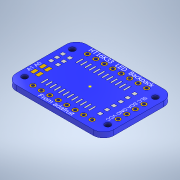
# Autodesk Inventor part: Part1
Saved by Autodesk Inventor 2021 (Build 250183000, 183)
## iProperties
Created: 2023-04-01
Part Number: Part1
Material: Generic
Document SubType Name: Modeling
Designer: stepa
Density: 1 g/cm^3
Appearance: Blue - Wall Paint - Glossy
Author: stepa
Autodesk Inventor part; units mm, degrees
ref_plane "YZ Plane" through (0, 0, 0) normal (1, 0, 0) x (0, 1, 0)
ref_plane "XZ Plane" through (0, 0, 0) normal (0, 1, 0) x (-1, 0, 0)
ref_plane "XY Plane" through (0, 0, 0) normal (0, 0, 1) x (1, 0, 0)
sketch "Sketch1" plane through (0, 0, 0) normal (0, 1, 0) x (-1, 0, 0)
  line L0 (11.15, -10.2) -> (-11.15, -10.2)
  line L1 (-14.15, -7.2) -> (-14.15, 7.2)
  line L2 (-11.15, 10.2) -> (11.15, 10.2)
  line L3 (14.15, 7.2) -> (14.15, -7.2)
  line L4 (14.15, -10.2) -> (-14.15, 10.2) construction
  line L5 (-14.15, -10.2) -> (14.15, 10.2) construction
  arc A0 (14.15, 7.2) -> (11.15, 10.2) centre (11.15, 7.2) ccw
  arc A1 (11.15, -10.2) -> (14.15, -7.2) centre (11.15, -7.2) ccw
  arc A2 (-14.15, -7.2) -> (-11.15, -10.2) centre (-11.15, -7.2) ccw
  arc A3 (-11.15, 10.2) -> (-14.15, 7.2) centre (-11.15, 7.2) ccw
  circle A4 centre (12.05, 6.9) radius 0.85
  circle A5 centre (12.05, -6.9) radius 0.85
  line L6 (0, 0) -> (0, 6.05)
  circle A6 centre (-12.05, 6.9) radius 0.85
  circle A7 centre (-12.05, -6.9) radius 0.85
  circle A8 centre (8.65, 7.9) radius 0.4
  circle A9 centre (6.2, 7.9) radius 0.4
  circle A10 centre (3.75, 7.9) radius 0.4
  circle A11 centre (1.3, 7.9) radius 0.4
  circle A12 centre (-1.15, 7.9) radius 0.4
  circle A13 centre (-3.6, 7.9) radius 0.4
  circle A14 centre (-6.05, 7.9) radius 0.4
  circle A15 centre (-8.5, 7.9) radius 0.4
  line L7 (0, 0) -> (3.75, 0)
  circle A16 centre (8.65, -7.9) radius 0.4
  circle A17 centre (6.2, -7.9) radius 0.4
  circle A18 centre (3.75, -7.9) radius 0.4
  circle A19 centre (1.3, -7.9) radius 0.4
  circle A20 centre (-1.15, -7.9) radius 0.4
  circle A21 centre (-3.6, -7.9) radius 0.4
  circle A22 centre (-6.05, -7.9) radius 0.4
  circle A23 centre (-8.5, -7.9) radius 0.4
  circle A24 centre (-12.15, 4) radius 0.4
  circle A25 centre (-12.15, 1.5) radius 0.4
  circle A26 centre (-12.15, -1) radius 0.4
  circle A27 centre (-12.15, -3.5) radius 0.4
  point P0 (0, -6.05)
  dimension "d0" = 20.4
  dimension "d1" = 28.3
  dimension "d2" = 3
  dimension "d3" = 1.7
  dimension "d4" = 1.7
  dimension "d5" = 3.3
  dimension "d6" = 3.3
  dimension "d7" = 2.1
  dimension "d8" = 2.1
  dimension "d9" = 0.8
  dimension "d10" = 5.5
  dimension "d11" = 2.3
  dimension "d14" = 2.45
  dimension "d19" = 0.8
  dimension "d20" = 2
  dimension "d21" = 2.5
  dimension "d22" = 6.2
  dimension "d23" = 0.8
  dimension "d24" = 2.5
  dimension "d25" = 0.8
  dimension "d26" = 0.8
  dimension "d27" = 2.5
  constraints: 28 centre point, 16 end point, 11 symmetric about line, 8 point on circle, 8 point on line, 8 tangent, 3 equal radius, 3 horizontal, 2 midpoint, 2 parallel, 1 perpendicular, 1 vertical, 24 other
  measures "d0" distance between parallel lines of L0 L2
  measures "d1" distance between parallel lines of L1 L3
  measures "d2" radius of A0
  measures "d3" diameter of A4
  measures "d4" diameter of A5
  measures "d5" distance from line of L0 A5.centre
  measures "d6" distance from line of L2 A4.centre
  measures "d7" distance from line of L3 A4.centre
  measures "d8" horizontal distance of L3.end A5.centre
  measures "d9" diameter of A8
  measures "d10" distance from line of L3 A8.centre
  measures "d11" distance from line of A8.centre L2
  measures "d14" distance of A8.centre A9.centre
  measures "d19" diameter of A24
  measures "d20" distance from line of L1 A24.centre
  measures "d21" distance of A24.centre A25.centre
  measures "d22" vertical distance of L2.start A24.centre
  measures "d23" diameter of A26
  measures "d24" distance of A25.centre A26.centre
  measures "d25" diameter of A27
  measures "d26" diameter of A25
  measures "d27" distance of A26.centre A27.centre
extrude "Extrusion1" add sketch "Sketch1" along normal mid plane 1.5
sketch "Sketch2" plane through (0, 0.75, 0) normal (0, 1, 0) x (1, 0, 0)
  line L0 (-11.15, -10.2) -> (11.15, -10.2) projected
  arc A0 (11.15, -10.2) -> (14.15, -7.2) centre (11.15, -7.2) ccw projected
  line L1 (14.15, -7.2) -> (14.15, 7.2) projected
  arc A1 (14.15, 7.2) -> (11.15, 10.2) centre (11.15, 7.2) ccw projected
  line L2 (11.15, 10.2) -> (-11.15, 10.2) projected
  arc A2 (-11.15, 10.2) -> (-14.15, 7.2) centre (-11.15, 7.2) ccw projected
  line L3 (-14.15, 7.2) -> (-14.15, -7.2) projected
  arc A3 (-14.15, -7.2) -> (-11.15, -10.2) centre (-11.15, -7.2) ccw projected
  circle A4 centre (12.15, 3.5) radius 0.4 projected
  circle A5 centre (12.15, -1.5) radius 0.4 projected
  circle A6 centre (3.6, 7.9) radius 0.4 projected
  circle A7 centre (6.05, 7.9) radius 0.4 projected
  circle A8 centre (-1.3, 7.9) radius 0.4 projected
  circle A9 centre (-6.2, 7.9) radius 0.4 projected
  circle A10 centre (8.5, -7.9) radius 0.4 projected
  circle A11 centre (6.05, -7.9) radius 0.4 projected
  circle A12 centre (3.6, -7.9) radius 0.4 projected
  circle A13 centre (1.15, -7.9) radius 0.4 projected
  circle A14 centre (-1.3, -7.9) radius 0.4 projected
  circle A15 centre (-3.75, -7.9) radius 0.4 projected
  circle A16 centre (-6.2, -7.9) radius 0.4 projected
  circle A17 centre (-8.65, -7.9) radius 0.4 projected
  circle A18 centre (-8.65, 7.9) radius 0.4 projected
  circle A19 centre (-3.75, 7.9) radius 0.4 projected
  circle A20 centre (1.15, 7.9) radius 0.4 projected
  circle A21 centre (8.5, 7.9) radius 0.4 projected
  circle A22 centre (12.15, -4) radius 0.4 projected
  circle A23 centre (12.15, 1) radius 0.4 projected
  circle A24 centre (12.05, 6.9) radius 0.85 projected
  circle A25 centre (12.05, -6.9) radius 0.85 projected
  circle A26 centre (-12.05, 6.9) radius 0.85 projected
  circle A27 centre (-12.05, -6.9) radius 0.85 projected
  circle A28 centre (-8.65, -7.9) radius 0.4 projected
  circle A29 centre (-8.65, -7.9) radius 0.75
  circle A30 centre (-6.2, -7.9) radius 0.4 projected
  circle A31 centre (-6.2, -7.9) radius 0.75
  circle A32 centre (-3.75, -7.9) radius 0.4 projected
  circle A33 centre (-3.75, -7.9) radius 0.75
  circle A34 centre (-1.3, -7.9) radius 0.4 projected
  circle A35 centre (-1.3, -7.9) radius 0.75
  circle A36 centre (1.15, -7.9) radius 0.4 projected
  circle A37 centre (1.15, -7.9) radius 0.75
  circle A38 centre (3.6, -7.9) radius 0.4 projected
  circle A39 centre (3.6, -7.9) radius 0.75
  circle A40 centre (6.05, -7.9) radius 0.4 projected
  circle A41 centre (6.05, -7.9) radius 0.75
  circle A42 centre (8.5, -7.9) radius 0.4 projected
  circle A43 centre (8.5, -7.9) radius 0.75
  circle A44 centre (12.15, -4) radius 0.4 projected
  circle A45 centre (12.15, -4) radius 0.75
  circle A46 centre (12.15, -1.5) radius 0.4 projected
  circle A47 centre (12.15, -1.5) radius 0.75
  circle A48 centre (12.15, 1) radius 0.4 projected
  circle A49 centre (12.15, 1) radius 0.75
  circle A50 centre (12.15, 3.5) radius 0.4 projected
  circle A51 centre (12.15, 3.5) radius 0.75
  circle A52 centre (8.5, 7.9) radius 0.4 projected
  circle A53 centre (8.5, 7.9) radius 0.75
  circle A54 centre (6.05, 7.9) radius 0.4 projected
  circle A55 centre (6.05, 7.9) radius 0.75
  circle A56 centre (3.6, 7.9) radius 0.4 projected
  circle A57 centre (3.6, 7.9) radius 0.75
  circle A58 centre (1.15, 7.9) radius 0.4 projected
  circle A59 centre (1.15, 7.9) radius 0.75
  circle A60 centre (-1.3, 7.9) radius 0.4 projected
  circle A61 centre (-1.3, 7.9) radius 0.75
  circle A62 centre (-3.75, 7.9) radius 0.4 projected
  circle A63 centre (-3.75, 7.9) radius 0.75
  circle A64 centre (-6.2, 7.9) radius 0.4 projected
  circle A65 centre (-6.2, 7.9) radius 0.75
  circle A66 centre (-8.65, 7.9) radius 0.75
  point P0 (0, 0)
  dimension "d30" = 1.5
  dimension "d31" = 1.5
  dimension "d32" = 1.5
  constraints: 20 centre point, 20 coincident
  measures "d30" diameter of A29
  measures "d31" diameter of A31
  measures "d32" diameter of A33
extrude "Extrusion2" cut sketch "Sketch2" against normal blind 0.001 contours A4 | A5 | A6 | A7 | A8 | A9 | A10 | A11 | A12 | A13 | A14 | A15 | A16 | A17 | A18 | A19 | A20 | A21 | A22 | A23 | A29 | A31 | A33 | A35 | A37 | A39 | A41 | A43 | A45 | A47 | A49 | A51 | A53 | A55 | A57 | A59 | A61 | A63 | A65 | A66
sketch "Sketch3" plane through (0, 0.75, 0) normal (0, 1, 0) x (1, 0, 0)
  line L0 (-12.55, -4.9) -> (-11.55, -4.9)
  line L1 (-11.55, -4.9) -> (-11.55, -3.3)
  line L2 (-11.55, -3.3) -> (-12.55, -3.3)
  line L3 (-12.55, -3.3) -> (-12.55, -4.9)
  line L4 (-12.55, -4.9) -> (-11.55, -3.3) construction
  line L5 (-11.55, -4.9) -> (-12.55, -3.3) construction
  line L6 (-14.15, 7.2) -> (-14.15, -7.2) projected
  line L7 (-11.15, -10.2) -> (11.15, -10.2) projected
  line L8 (-11.05, -4.9) -> (-10.05, -4.9)
  line L9 (-10.05, -4.9) -> (-10.05, -3.3)
  line L10 (-10.05, -3.3) -> (-11.05, -3.3)
  line L11 (-11.05, -3.3) -> (-11.05, -4.9)
  line L12 (-11.05, -4.9) -> (-10.05, -3.3) construction
  line L13 (-10.05, -4.9) -> (-11.05, -3.3) construction
  line L14 (-12.55, -2.4) -> (-11.55, -2.4)
  line L15 (-11.55, -2.4) -> (-11.55, -0.8)
  line L16 (-11.55, -0.8) -> (-12.55, -0.8)
  line L17 (-12.55, -0.8) -> (-12.55, -2.4)
  line L18 (-12.55, -2.4) -> (-11.55, -0.8) construction
  line L19 (-11.55, -2.4) -> (-12.55, -0.8) construction
  line L20 (-11.05, -2.4) -> (-10.05, -2.4)
  line L21 (-10.05, -2.4) -> (-10.05, -0.8)
  line L22 (-10.05, -0.8) -> (-11.05, -0.8)
  line L23 (-11.05, -0.8) -> (-11.05, -2.4)
  line L24 (-11.05, -2.4) -> (-10.05, -0.8) construction
  line L25 (-10.05, -2.4) -> (-11.05, -0.8) construction
  point P0 (0, 0)
  point P1 (-12.05, -4.1)
  point P2 (-10.55, -4.1)
  point P3 (-12.05, -1.6)
  point P4 (-10.55, -1.6)
  dimension "d35" = 1.6
  dimension "d36" = 1.6
  dimension "d37" = 1
  dimension "d38" = 5.3
  dimension "d41" = 1.5
  dimension "d44" = 2.5
  constraints: 48 end point, 8 midpoint, 2 collinear, 2 horizontal, 2 parallel, 1 perpendicular, 1 vertical, 31 other
  measures "d35" distance of L2.end L0.start
  measures "d36" distance between parallel lines of L6 L3
  measures "d37" distance of L1.end L2.end
  measures "d38" distance between parallel lines of L7 L0
  measures "d41" distance of L0.start L8.start
  measures "d44" distance of L0.start L14.start
extrude "Extrusion3" cut sketch "Sketch3" against normal blind 0.001
sketch "Sketch4" plane through (0, 0.75, 0) normal (0, 1, 0) x (1, 0, 0)
  line L0 (-5.456, -8.6683) -> (16.4652, -8.6683) construction
  line L1 (16.4652, -8.6683) -> (16.4652, 6.2441) construction
  line L2 (16.4652, 6.2441) -> (-5.456, 6.2441) construction
  line L3 (-5.456, 6.2441) -> (-5.456, -8.6683) construction
  line L4 (-13.845, -4.8059) -> (-13.845, 1.6171) construction
  line L5 (-13.845, 1.6171) -> (-10.9674, 1.6171) construction
  line L6 (-10.9674, 1.6171) -> (-10.9674, -4.8059) construction
  line L7 (-10.9674, -4.8059) -> (-13.845, -4.8059) construction
  line L8 (11.2525, 5.5942) -> (11.2525, -7.2168) construction
  line L9 (11.2525, -7.2168) -> (7.828, -7.2168) construction
  line L10 (7.828, -7.2168) -> (7.828, 5.5942) construction
  line L11 (7.828, 5.5942) -> (11.2525, 5.5942) construction
  line L12 (-9.4713, 10.0949) -> (13.4648, 10.0949) construction
  line L13 (13.4648, 10.0949) -> (13.4648, -4.2973) construction
  line L14 (13.4648, -4.2973) -> (-9.4713, -4.2973) construction
  line L15 (-9.4713, -4.2973) -> (-9.4713, 10.0949) construction
  point P0 (0, 0)
  dimension "d0" = 20.4
  dimension "d1" = 28.3
  dimension "d2" = 3
  dimension "d3" = 1.7
  dimension "d4" = 1.7
  dimension "d5" = 3.3
  dimension "d6" = 3.3
  dimension "d7" = 2.1
  dimension "d8" = 2.1
  dimension "d9" = 0.8
  dimension "d10" = 5.5
  dimension "d11" = 2.3
  dimension "d14" = 2.45
  dimension "d19" = 0.8
  dimension "d20" = 2
  dimension "d21" = 2.5
  dimension "d22" = 6.2
  dimension "d23" = 0.8
  dimension "d24" = 2.5
  dimension "d25" = 0.8
  dimension "d26" = 0.8
  dimension "d27" = 2.5
  constraints: 8 other
sketch "Sketch5" plane through (0, 0.75, 0) normal (0, 1, 0) x (1, 0, 0)
  line L0 (7.65, -5.7) -> (8.65, -5.7)
  line L1 (8.65, -5.7) -> (8.65, -4.7)
  line L2 (8.65, -4.7) -> (7.65, -4.7)
  line L3 (7.65, -4.7) -> (7.65, -5.7)
  line L4 (-11.15, -10.2) -> (11.15, -10.2) projected
  line L5 (14.15, -7.2) -> (14.15, 7.2) projected
  line L6 (7.65, -2.7) -> (7.65, -3.7)
  line L7 (7.65, -3.7) -> (8.65, -3.7)
  line L8 (8.65, -3.7) -> (8.65, -2.7)
  line L9 (8.65, -2.7) -> (7.65, -2.7)
  line L10 (7.65, 1.3) -> (7.65, 0.3)
  line L11 (7.65, -0.7) -> (7.65, -1.7)
  line L12 (7.65, 0.3) -> (8.65, 0.3)
  line L13 (7.65, -1.7) -> (8.65, -1.7)
  line L14 (8.65, 1.3) -> (7.65, 1.3)
  line L15 (8.65, -0.7) -> (7.65, -0.7)
  line L16 (8.65, -1.7) -> (8.65, -0.7)
  line L17 (8.65, 0.3) -> (8.65, 1.3)
  line L18 (7.65, 5.3) -> (7.65, 4.3)
  line L19 (7.65, 3.3) -> (7.65, 2.3)
  line L20 (7.65, 4.3) -> (8.65, 4.3)
  line L21 (7.65, 2.3) -> (8.65, 2.3)
  line L22 (8.65, 5.3) -> (7.65, 5.3)
  line L23 (8.65, 3.3) -> (7.65, 3.3)
  line L24 (8.65, 2.3) -> (8.65, 3.3)
  line L25 (8.65, 4.3) -> (8.65, 5.3)
  line L26 (-12.75, 0.4818) -> (-11.75, 0.4818)
  line L27 (-11.75, 0.4818) -> (-11.75, 1.4818)
  line L28 (-11.75, 1.4818) -> (-12.75, 1.4818)
  line L29 (-12.75, 1.4818) -> (-12.75, 0.4818)
  line L30 (-10.75, 0.4818) -> (-9.75, 0.4818)
  line L31 (-9.75, 0.4818) -> (-9.75, 1.4818)
  line L32 (-9.75, 1.4818) -> (-10.75, 1.4818)
  line L33 (-10.75, 1.4818) -> (-10.75, 0.4818)
  line L34 (-14.15, 7.2) -> (-14.15, -7.2) projected
  line L35 (-9.75, 2.1818) -> (-9.75, 3.1818)
  line L36 (-9.75, 3.1818) -> (-10.75, 3.1818)
  line L37 (-10.75, 2.1818) -> (-9.75, 2.1818)
  line L38 (-10.75, 3.1818) -> (-10.75, 2.1818)
  line L39 (-11.75, 2.1818) -> (-11.75, 3.1818)
  line L40 (-11.75, 3.1818) -> (-12.75, 3.1818)
  line L41 (-12.75, 2.1818) -> (-11.75, 2.1818)
  line L42 (-12.75, 3.1818) -> (-12.75, 2.1818)
  line L43 (-9.75, 3.8818) -> (-9.75, 4.8818)
  line L44 (-9.75, 4.8818) -> (-10.75, 4.8818)
  line L45 (-10.75, 3.8818) -> (-9.75, 3.8818)
  line L46 (-10.75, 4.8818) -> (-10.75, 3.8818)
  line L47 (-11.75, 3.8818) -> (-11.75, 4.8818)
  line L48 (-11.75, 4.8818) -> (-12.75, 4.8818)
  line L49 (-12.75, 3.8818) -> (-11.75, 3.8818)
  line L50 (-12.75, 4.8818) -> (-12.75, 3.8818)
  line L51 (-8.3157, -6.0644) -> (-7.8657, -6.0644)
  line L52 (-7.8657, -6.0644) -> (-7.8657, -4.0644)
  line L53 (-7.8657, -4.0644) -> (-8.3157, -4.0644)
  line L54 (-8.3157, -4.0644) -> (-8.3157, -6.0644)
  line L55 (-6.6157, -4.0644) -> (-7.0657, -4.0644)
  line L56 (-7.0657, -4.0644) -> (-7.0657, -6.0644)
  line L57 (-7.0657, -6.0644) -> (-6.6157, -6.0644)
  line L58 (-6.6157, -6.0644) -> (-6.6157, -4.0644)
  line L59 (-5.3657, -4.0644) -> (-5.8157, -4.0644)
  line L60 (-5.8157, -4.0644) -> (-5.8157, -6.0644)
  line L61 (-5.8157, -6.0644) -> (-5.3657, -6.0644)
  line L62 (-5.3657, -6.0644) -> (-5.3657, -4.0644)
  line L63 (-4.1157, -4.0644) -> (-4.5657, -4.0644)
  line L64 (-4.5657, -4.0644) -> (-4.5657, -6.0644)
  line L65 (-4.5657, -6.0644) -> (-4.1157, -6.0644)
  line L66 (-4.1157, -6.0644) -> (-4.1157, -4.0644)
  line L67 (-2.8657, -4.0644) -> (-3.3157, -4.0644)
  line L68 (-3.3157, -4.0644) -> (-3.3157, -6.0644)
  line L69 (-3.3157, -6.0644) -> (-2.8657, -6.0644)
  line L70 (-2.8657, -6.0644) -> (-2.8657, -4.0644)
  line L71 (-1.6157, -4.0644) -> (-2.0657, -4.0644)
  line L72 (-2.0657, -4.0644) -> (-2.0657, -6.0644)
  line L73 (-2.0657, -6.0644) -> (-1.6157, -6.0644)
  line L74 (-1.6157, -6.0644) -> (-1.6157, -4.0644)
  line L75 (-0.3657, -4.0644) -> (-0.8157, -4.0644)
  line L76 (-0.8157, -4.0644) -> (-0.8157, -6.0644)
  line L77 (-0.8157, -6.0644) -> (-0.3657, -6.0644)
  line L78 (-0.3657, -6.0644) -> (-0.3657, -4.0644)
  line L79 (0.8843, -4.0644) -> (0.4343, -4.0644)
  line L80 (0.4343, -4.0644) -> (0.4343, -6.0644)
  line L81 (0.4343, -6.0644) -> (0.8843, -6.0644)
  line L82 (0.8843, -6.0644) -> (0.8843, -4.0644)
  line L83 (2.1343, -4.0644) -> (1.6843, -4.0644)
  line L84 (1.6843, -4.0644) -> (1.6843, -6.0644)
  line L85 (1.6843, -6.0644) -> (2.1343, -6.0644)
  line L86 (2.1343, -6.0644) -> (2.1343, -4.0644)
  line L87 (3.3843, -4.0644) -> (2.9343, -4.0644)
  line L88 (2.9343, -4.0644) -> (2.9343, -6.0644)
  line L89 (2.9343, -6.0644) -> (3.3843, -6.0644)
  line L90 (3.3843, -6.0644) -> (3.3843, -4.0644)
  line L91 (4.6343, -4.0644) -> (4.1843, -4.0644)
  line L92 (4.1843, -4.0644) -> (4.1843, -6.0644)
  line L93 (4.1843, -6.0644) -> (4.6343, -6.0644)
  line L94 (4.6343, -6.0644) -> (4.6343, -4.0644)
  line L95 (5.8843, -4.0644) -> (5.4343, -4.0644)
  line L96 (5.4343, -4.0644) -> (5.4343, -6.0644)
  line L97 (5.4343, -6.0644) -> (5.8843, -6.0644)
  line L98 (5.8843, -6.0644) -> (5.8843, -4.0644)
  line L99 (0, 0) -> (-2.4399, 0)
  line L100 (-8.3157, 6.0644) -> (-7.8657, 6.0644)
  line L101 (-7.8657, 6.0644) -> (-7.8657, 4.0644)
  line L102 (-7.8657, 4.0644) -> (-8.3157, 4.0644)
  line L103 (-8.3157, 4.0644) -> (-8.3157, 6.0644)
  line L104 (-6.6157, 4.0644) -> (-7.0657, 4.0644)
  line L105 (-7.0657, 4.0644) -> (-7.0657, 6.0644)
  line L106 (-7.0657, 6.0644) -> (-6.6157, 6.0644)
  line L107 (-6.6157, 6.0644) -> (-6.6157, 4.0644)
  line L108 (-5.3657, 4.0644) -> (-5.8157, 4.0644)
  line L109 (-5.8157, 4.0644) -> (-5.8157, 6.0644)
  line L110 (-5.8157, 6.0644) -> (-5.3657, 6.0644)
  line L111 (-5.3657, 6.0644) -> (-5.3657, 4.0644)
  line L112 (-4.1157, 4.0644) -> (-4.5657, 4.0644)
  line L113 (-4.5657, 4.0644) -> (-4.5657, 6.0644)
  line L114 (-4.5657, 6.0644) -> (-4.1157, 6.0644)
  line L115 (-4.1157, 6.0644) -> (-4.1157, 4.0644)
  line L116 (-2.8657, 4.0644) -> (-3.3157, 4.0644)
  line L117 (-3.3157, 4.0644) -> (-3.3157, 6.0644)
  line L118 (-3.3157, 6.0644) -> (-2.8657, 6.0644)
  line L119 (-2.8657, 6.0644) -> (-2.8657, 4.0644)
  line L120 (-1.6157, 4.0644) -> (-2.0657, 4.0644)
  line L121 (-2.0657, 4.0644) -> (-2.0657, 6.0644)
  line L122 (-2.0657, 6.0644) -> (-1.6157, 6.0644)
  line L123 (-1.6157, 6.0644) -> (-1.6157, 4.0644)
  line L124 (-0.3657, 4.0644) -> (-0.8157, 4.0644)
  line L125 (-0.8157, 4.0644) -> (-0.8157, 6.0644)
  line L126 (-0.8157, 6.0644) -> (-0.3657, 6.0644)
  line L127 (-0.3657, 6.0644) -> (-0.3657, 4.0644)
  line L128 (0.8843, 4.0644) -> (0.4343, 4.0644)
  line L129 (0.4343, 4.0644) -> (0.4343, 6.0644)
  line L130 (0.4343, 6.0644) -> (0.8843, 6.0644)
  line L131 (0.8843, 6.0644) -> (0.8843, 4.0644)
  line L132 (2.1343, 4.0644) -> (1.6843, 4.0644)
  line L133 (1.6843, 4.0644) -> (1.6843, 6.0644)
  line L134 (1.6843, 6.0644) -> (2.1343, 6.0644)
  line L135 (2.1343, 6.0644) -> (2.1343, 4.0644)
  line L136 (3.3843, 4.0644) -> (2.9343, 4.0644)
  line L137 (2.9343, 4.0644) -> (2.9343, 6.0644)
  line L138 (2.9343, 6.0644) -> (3.3843, 6.0644)
  line L139 (3.3843, 6.0644) -> (3.3843, 4.0644)
  line L140 (4.6343, 4.0644) -> (4.1843, 4.0644)
  line L141 (4.1843, 4.0644) -> (4.1843, 6.0644)
  line L142 (4.1843, 6.0644) -> (4.6343, 6.0644)
  line L143 (4.6343, 6.0644) -> (4.6343, 4.0644)
  line L144 (5.8843, 4.0644) -> (5.4343, 4.0644)
  line L145 (5.4343, 4.0644) -> (5.4343, 6.0644)
  line L146 (5.4343, 6.0644) -> (5.8843, 6.0644)
  line L147 (5.8843, 6.0644) -> (5.8843, 4.0644)
  dimension "d49" = 1
  dimension "d50" = 1
  dimension "d51" = 4.5
  dimension "d52" = 5.5
  dimension "d55" = 2
  dimension "d62" = 4
  dimension "d67" = 1
  dimension "d68" = 1
  dimension "d69" = 1
  dimension "d70" = 1
  dimension "d71" = 1.4
  dimension "d72" = 1
  dimension "d75" = 1.7
  dimension "d80" = 2
  dimension "d81" = 0.45
  dimension "d84" = 1.25
  constraints: 290 end point, 48 symmetric about line, 8 parallel, 6 horizontal, 4 collinear, 4 perpendicular, 3 point on line, 3 vertical, 156 other
  measures "d49" distance of L2.end L0.start
  measures "d50" distance of L1.end L2.end
  measures "d51" distance between parallel lines of L4 L0
  measures "d52" distance between parallel lines of L5 L1
  measures "d55" distance of L0.start L6.end
  measures "d62" distance of L6.end L10.end
  measures "d67" distance of L28.end L26.start
  measures "d68" distance of L27.end L28.end
  measures "d69" distance of L32.end L30.start
  measures "d70" distance of L31.end L32.end
  measures "d71" distance between parallel lines of L34 L29
  measures "d72" distance between parallel lines of L33 L27
  measures "d75" distance of L31.end L35.end
  measures "d80" distance of L53.end L51.start
  measures "d81" distance between parallel lines of L54 L52
  measures "d84" distance of L53.end L55.end
extrude "Extrusion4" cut sketch "Sketch5" against normal blind 0.001
mirror "Mirror1" about plane through (0, 0, 0) normal (0, 1, 0) of "Extrusion2"
body "Solid1"
